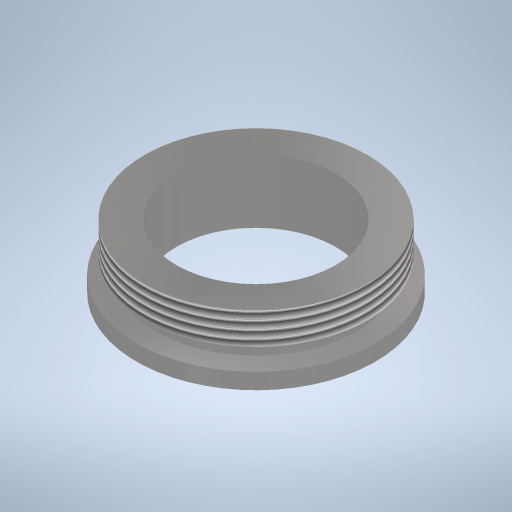
# Autodesk Inventor part: 034
Saved by Autodesk Inventor 2023 (Build 270158000, 158)
## iProperties
Created: 2022-04-18
Part Number: 034
Material: Stainless Steel, Austenitic
Document SubType Name: Modeling
Designer: vmiguel
Density: 8 g/cm^3
Appearance: Semi-Polished
Author: vmiguel
Autodesk Inventor part; units mm, degrees
ref_plane "YZ Plane" through (0, 0, 0) normal (1, 0, 0) x (0, 1, 0)
ref_plane "XZ Plane" through (0, 0, 0) normal (0, 1, 0) x (-1, 0, 0)
ref_plane "XY Plane" through (0, 0, 0) normal (0, 0, 1) x (1, 0, 0)
sketch "Sketch1" plane through (0, 0, 0) normal (1, 0, 0) x (0, 1, 0)
  line L0 (0, 0) -> (7.3009, 0)
  line L1 (0, -10) -> (8, -10)
  line L2 (0, -10) -> (0, -15)
  line L3 (0, -15) -> (2, -15)
  line L4 (2, -15) -> (2, -14)
  line L5 (2, -14) -> (8, -14)
  line L6 (8, -14) -> (8, -10)
  line L7 (2, -14) -> (2, -12.5)
  line L8 (2, -12.5) -> (4, -12.5)
  line L9 (4, -12.5) -> (4, -14)
  point P0 (4, -10)
  dimension "d0" = 20
  dimension "d1" = 6
  dimension "d2" = 2
  dimension "d3" = 28
  dimension "d4" = 30
  dimension "d8" = 2
  dimension "d9" = 1.5
  constraints: 20 end point, 6 perpendicular, 2 horizontal, 2 vertical, 1 midpoint, 1 point on line, 1 vertical alignment
  measures "d0" diameter of point (4, -10) L0
  measures "d1" distance of L4.end L5.end
  measures "d2" distance of L2.end L3.end
  measures "d3" diameter of L5 L0
  measures "d4" diameter of L3 L0
  measures "d8" distance of L7.end L8.end
  measures "d9" distance of L8.end L9.end
revolve "Revolution1" add sketch "Sketch1" angle 360 about axis through (0, 0, 0) along (0, 1, 0) contours L1 L6 L5 L9 L8 L7 L4 L3 L2
thread "Thread1" size "M28x1" class "6g" standard "ANSI Metric M Profile" full length
body "Solid1"
